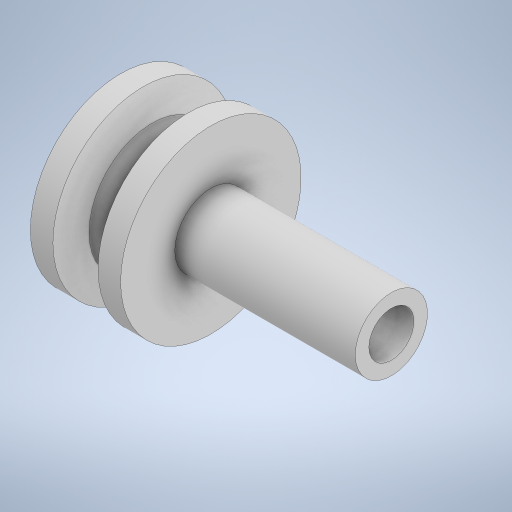
# Autodesk Inventor part: Шкив 20
Saved by Autodesk Inventor 2023 (Build 270158000, 158)
## iProperties
Created: 2022-05-01
Part Number: Шкив 20
Material: Типовые
Document SubType Name: Modeling
Designer: User
Density: 1 g/cm^3
Appearance: По умолчанию
Author: User
Autodesk Inventor part; units mm, degrees
ref_plane "YZ Plane" through (0, 0, 0) normal (1, 0, 0) x (0, 1, 0)
ref_plane "XZ Plane" through (0, 0, 0) normal (0, 1, 0) x (-1, 0, 0)
ref_plane "XY Plane" through (0, 0, 0) normal (0, 0, 1) x (1, 0, 0)
sketch "Эскиз1" plane through (0, 0, 0) normal (0, 1, 0) x (-1, 0, 0)
  line L0 (0, 20) -> (20, 20)
  line L1 (20, 20) -> (20, 0)
  line L2 (20, 0) -> (0, 0)
  line L3 (20, 20) -> (13, 20)
  line L4 (13, 20) -> (13, 14)
  line L5 (13, 14) -> (7, 14)
  line L6 (7, 14) -> (7, 20)
  line L7 (20, 0) -> (-40, 0)
  line L8 (-40, 0) -> (-40, 8)
  line L9 (-40, 8) -> (0, 8)
  line L10 (-40, 0) -> (-40, 5)
  line L11 (-40, 5) -> (20, 5)
  line L12 (0, 0) -> (0, 5)
  line L13 (0, 8) -> (0, 20)
  dimension "d0" = 20
  dimension "d1" = 20
  dimension "d2" = 7
  dimension "d3" = 6
  dimension "d4" = 6
  dimension "d5" = 60
  dimension "d6" = 8
  dimension "d7" = 5
  constraints: 28 end point, 12 perpendicular, 5 point on line, 2 vertical
  measures "d0" distance of L2.end L0.start
  measures "d1" distance of L0.start L0.end
  measures "d2" distance of L0.end L3.end
  measures "d3" distance of L3.end L4.end
  measures "d4" distance of L4.end L5.end
  measures "d5" distance of L1.end L7.end
  measures "d6" distance of L7.end L8.end
  measures "d7" distance of L7.end L10.end
revolve "Вращение1" add sketch "Эскиз1" angle 360 about axis through (-20, 0, 0) along (1, 0, 0) contours L0 L6 L5 L4 L1 L11 L8 L9 L13
chamfer "Фаска1" distance 6 distance2 2 1 edges at (-13, 0, -20) measured on face at (-13, 0, -19.5)
chamfer "Фаска2" distance 2 distance2 6 1 edges at (-7, 0, -20) measured on face at (-6.5, 0, -20)
